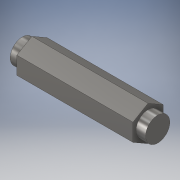
# Autodesk Inventor part: Shaft Jr
Saved by Autodesk Inventor 2019.4 (Build 234330000, 330)
## iProperties
Created: 2019-12-11
Part Number: Shaft Jr
Material: Steel, Mild
Document SubType Name: Modeling
Designer: admin
Density: 7.85 g/cm^3
Appearance: Semi-Polished
Author: admin
Autodesk Inventor part; units mm, degrees
ref_plane "YZ Plane" through (0, 0, 0) normal (1, 0, 0) x (0, 1, 0)
ref_plane "XZ Plane" through (0, 0, 0) normal (0, 1, 0) x (-1, 0, 0)
ref_plane "XY Plane" through (0, 0, 0) normal (0, 0, 1) x (1, 0, 0)
sketch "Sketch1" plane through (0, 0, 0) normal (0, 0, 1) x (1, 0, 0)
  line L0 (0, 0) -> (0, 5)
  line L1 (0, 5) -> (4, 5)
  line L2 (4, 5) -> (4, 15)
  line L3 (4, 15) -> (52, 15)
  line L4 (52, 15) -> (52, 5)
  line L5 (52, 5) -> (56, 5)
  line L6 (56, 5) -> (56, 0)
  line L7 (56, 0) -> (0, 0)
  dimension "d0" = 5
  dimension "d1" = 15
  dimension "d2" = 4
  dimension "d3" = 4
  dimension "d4" = 48
  constraints: 16 end point, 6 perpendicular, 2 point on line, 1 vertical
  measures "d0" distance of L5.end L6.end
  measures "d1" distance between parallel lines of L7 L3
  measures "d2" distance of L0.end L1.end
  measures "d3" distance of L4.end L5.end
  measures "d4" distance of L2.end L3.end
revolve "Revolution1" add sketch "Sketch1" angle 360 about axis through (56, 0, 0) along (-1, 0, 0)
sketch "Sketch2" plane through (52, 0, 0) normal (1, 0, 0) x (0, 0, -1)
  line L0 (0, 7.2169) -> (6.25, 3.6084)
  line L1 (6.25, 3.6084) -> (6.25, -3.6084)
  line L2 (6.25, -3.6084) -> (0, -7.2169)
  line L3 (0, -7.2169) -> (-6.25, -3.6084)
  line L4 (-6.25, -3.6084) -> (-6.25, 3.6084)
  line L5 (-6.25, 3.6084) -> (0, 7.2169)
  circle A0 centre (0, 0) radius 15 projected
  dimension "d6" = 12.5
  constraints: 12 end point, 1 coincident, 13 other
  measures "d6" distance between parallel lines of L1 L4
extrude "Extrusion1" cut sketch "Sketch2" against normal through all
body "Solid1"
